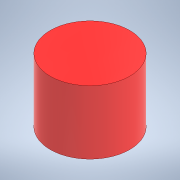
# Autodesk Inventor part: motor-mount-top
Saved by Autodesk Inventor 2021 (Build 250183000, 183)
## iProperties
Created: 2021-03-30
Part Number: motor-mount-top
Material: ABS Plastic
Document SubType Name: Modeling
Designer: samlo
Density: 1.06 g/cm^3
Appearance: Light Red
Author: samlo
Autodesk Inventor part; units mm, degrees
ref_plane "YZ Plane" through (0, 0, 0) normal (1, 0, 0) x (0, 1, 0)
ref_plane "XZ Plane" through (0, 0, 0) normal (0, 1, 0) x (-1, 0, 0)
ref_plane "XY Plane" through (0, 0, 0) normal (0, 0, 1) x (1, 0, 0)
sketch "Sketch1" plane through (0, 0, 0) normal (0, 0, 1) x (1, 0, 0)
  line L0 (0, 40) -> (25, 40)
  line L1 (25, 40) -> (25, 0)
  line L2 (25, 0) -> (11.665, 0)
  line L3 (11.665, 0) -> (11.665, 20)
  line L4 (11.665, 20) -> (0, 20)
  line L5 (0, 20) -> (0, 40)
  point P0 (0, 0)
  dimension "d0" = 40
  dimension "d1" = 20
  dimension "d2" = 0
  dimension "d3" = 11.665
  dimension "d4" = 0
  dimension "d5" = 25
  constraints: 12 end point, 5 perpendicular, 1 horizontal
  measures "d0" distance of L0.end L1.end
  measures "d1" distance of L2.end L3.end
  measures "d2" vertical distance of L2.end point (0, 0)
  measures "d3" distance of L3.end L4.end
  measures "d4" horizontal distance of L4.end point (0, 0)
  measures "d5" distance of L0.start L0.end
revolve "Revolution1" add sketch "Sketch1" angle 360 about axis through (0, 20, 0) along (0, 1, 0)
body "Solid1"
